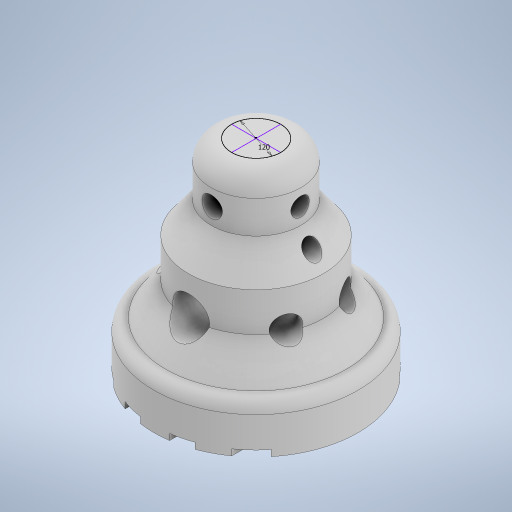
# Autodesk Inventor part: reef1
Saved by Autodesk Inventor 2024.3 (Build 283343000, 343)
## iProperties
Created: 2026-04-06
Part Number: reef1
Material: Genérico
Document SubType Name: Modeling
Designer: elena
Density: 1 g/cm^3
Appearance: Valor por defecto
Author: elena
Autodesk Inventor part; units mm, degrees
sketch "Boceto1" plane through (0, 0, 0) normal (0, 1, 0) x (-1, 0, 0)
  circle A0 centre (0, 0) radius 250
  dimension "d0" = 500
  constraints: 1 centre point, 1 coincident
  measures "d0" diameter of A0
extrude "Extrusión1" add sketch "Boceto1" along normal blind 100
sketch "Boceto2" plane through (0, 100, 0) normal (0, 1, 0) x (1, 0, 0)
  circle A0 centre (0, 0) radius 165
  dimension "d3" = 330
  constraints: 1 centre point, 1 coincident
  measures "d3" diameter of A0
extrude "Extrusión2" add sketch "Boceto2" along normal blind 175
chamfer "Chaflán1" distance 80 angle 35 1 edges at (-165, 100, 0) measured on face at (-165, 100.5, 0)
sketch "Boceto3" plane through (0, 275, 0) normal (0, 1, 0) x (1, 0, 0)
  point P0 (0, 0)
ref_plane "Plano de trabajo1" through (0, 350, 0) normal (0, 1, 0) x (1, 0, 0)
sketch "Boceto4" plane through (0, 350, 0) normal (0, 1, 0) x (1, 0, 0)
  circle A0 centre (0, 0) radius 110
  dimension "d10" = 220
  constraints: 1 centre point, 1 coincident
  measures "d10" diameter of A0
loft "Solevación1" add profiles "Boceto4" section 1 edges at (-165, 275, 0)
fillet "Empalme1" radius 30 1 edges at (250, 100, 0)
sketch "Boceto5" plane through (0, 350, 0) normal (0, 1, 0) x (1, 0, 0)
  circle A0 centre (0, 0) radius 110
  dimension "d16" = 220
  constraints: 1 centre point, 1 coincident
  measures "d16" diameter of A0
extrude "Extrusión3" add sketch "Boceto5" along normal blind 130
fillet "Empalme2" radius 50 1 edges at (-110, 480, 0)
sketch "Boceto6" plane through (0, 0, 0) normal (0, -1, 0) x (1, 0, 0)
  circle A0 centre (0, 0) radius 250
  dimension "d20" = 500
  constraints: 1 centre point, 1 coincident
  measures "d20" diameter of A0
extrude "Extrusión4" add sketch "Boceto6" along normal blind 20
sketch "Boceto7" plane through (0, 480, 0) normal (0, 1, 0) x (1, 0, 0)
  line L0 (-60.1732, 0) -> (60, 0)
  circle A0 centre (0, 0) radius 60 projected
  constraints: 2 end point, 1 horizontal, 1 horizontal alignment, 1 other
ref_plane "Plano de trabajo2" through (-60.1732, 480, 0) normal (0, 0, 1) x (1, 0, 0)
sketch "Boceto8" plane through (-60.1732, 480, 0) normal (0, 0, 1) x (1, 0, 0)
  point P0 (60.1732, -480)
sketch "Boceto9" plane through (0, -20, 0) normal (0, -1, 0) x (1, 0, 0)
  line L0 (0, 233.6633) -> (0, -235.8369)
  line L1 (-194.5383, 266.2675) -> (-194.5383, -277.679)
  line L2 (-194.5383, -277.679) -> (-144.5383, -277.679)
  line L3 (-144.5383, -277.679) -> (-144.5383, 266.2675)
  line L4 (-144.5383, 266.2675) -> (-194.5383, 266.2675)
  line L5 (-85.8577, 266.2675) -> (-85.8577, -277.679)
  line L6 (-85.8577, -277.679) -> (-35.8577, -277.679)
  line L7 (-35.8577, -277.679) -> (-35.8577, 266.2675)
  line L8 (-35.8577, 266.2675) -> (-85.8577, 266.2675)
  line L9 (194.5383, 266.2675) -> (194.5383, -277.679)
  line L10 (194.5383, -277.679) -> (144.5383, -277.679)
  line L11 (144.5383, -277.679) -> (144.5383, 266.2675)
  line L12 (144.5383, 266.2675) -> (194.5383, 266.2675)
  line L13 (85.8577, 266.2675) -> (85.8577, -277.679)
  line L14 (35.8577, -277.679) -> (35.8577, 266.2675)
  line L15 (85.8577, -277.679) -> (35.8577, -277.679)
  line L16 (35.8577, 266.2675) -> (85.8577, 266.2675)
  point P0 (0, 0)
  dimension "d24" = 50
  dimension "d25" = 50
  constraints: 34 end point, 8 symmetric about line, 4 perpendicular, 3 vertical, 2 horizontal
  measures "d24" distance of L1.end L2.end
  measures "d25" distance of L5.end L7.start
extrude "Extrusión5" cut sketch "Boceto9" against normal blind 15
sketch "Boceto10" plane through (-60.1732, 480, 0) normal (0, 0, 1) x (1, 0, 0)
  point P0 (60.1732, -480)
sketch "Boceto11" plane through (-60.1732, 480, 0) normal (0, 0, 1) x (1, 0, 0)
  circle A0 centre (60.1732, -292.5) radius 45
  point P0 (60.1732, -480)
  dimension "d28" = 90
  constraints: 1 centre point
  measures "d28" diameter of A0
extrude "Extrusión6" cut sketch "Boceto11" along normal mid plane 500
sketch "Boceto12" plane through (-60.1732, 480, 0) normal (0, 0, 1) x (1, 0, 0)
  line L0 (60.1732, -240.2586) -> (60.1732, -191.3822)
  line L1 (225.1732, -205) -> (-104.8268, -205) projected
  line L2 (225.1732, -300) -> (225.1732, -205) projected
  line L3 (225.1732, -300) -> (225.1732, -205)
  circle A0 centre (150.173, -292.5) radius 30
  line L4 (-104.8268, -300) -> (-104.8268, -205)
  circle A1 centre (-29.8267, -292.5) radius 30
  point P0 (60.1732, -480)
  dimension "d31" = 60
  constraints: 6 end point, 3 symmetric about line, 2 centre point, 2 point on line, 1 perpendicular, 1 other
  measures "d31" diameter of A0
revolve "Revolución1" cut sketch "Boceto12" angle 360 about axis through (-165, 180, 0) along (0, 1, 0) contours A1
revolve "Revolución2" cut sketch "Boceto12" angle 360 about axis through (165, 180, 0) along (0, 1, 0) contours A0
sketch "Boceto13" plane through (0, 480, 0) normal (0, 1, 0) x (1, 0, 0)
  circle A0 centre (0, 0) radius 60
  dimension "d34" = 120
  constraints: 1 centre point, 1 coincident
  measures "d34" diameter of A0
sketch "Boceto14" plane through (0, 480, 0) normal (0, 1, 0) x (1, 0, 0)
  circle A0 centre (0, 0) radius 60 projected
  line L0 (0, 60) -> (0, -60)
  constraints: 2 end point, 2 point on circle, 1 vertical
ref_plane "Plano de trabajo3" through (0, 480, -60) normal (-1, 0, 0) x (0, 0, 1)
sketch "Boceto15" plane through (-60.1732, 480, 0) normal (0, 0, 1) x (1, 0, 0)
  circle A0 centre (60.1732, -90) radius 25
  point P0 (60.1732, -480)
  dimension "d36" = 50
  constraints: 1 centre point
  measures "d36" diameter of A0
extrude "Extrusión7" cut sketch "Boceto15" along normal mid plane 500
sketch "Boceto16" plane through (0, 480, -60) normal (-1, 0, 0) x (0, 0, 1)
  circle A0 centre (60, -167.5) radius 20
  point P0 (60, -480)
  dimension "d39" = 40
  constraints: 1 centre point
  measures "d39" diameter of A0
extrude "Extrusión8" cut sketch "Boceto16" along normal mid plane 500
sketch "Boceto17" plane through (0, 480, -60) normal (-1, 0, 0) x (0, 0, 1)
  point P0 (60, -480)
ref_plane "Plano de trabajo4" through (-120, 480, -60) normal (-1, 0, 0) x (0, 0, 1)
sketch "Boceto18" plane through (-120, 480, -60) normal (-1, 0, 0) x (0, 0, 1)
  circle A0 centre (60, -90) radius 22.5
  point P0 (60, -480)
  dimension "d43" = 45
  constraints: 1 centre point
  measures "d43" diameter of A0
extrude "Extrusión9" cut sketch "Boceto18" against normal blind 60
ref_plane "Plano de trabajo5" through (120, 480, -60) normal (-1, 0, 0) x (0, 0, 1)
sketch "Boceto19" plane through (120, 480, -60) normal (-1, 0, 0) x (0, 0, 1)
  circle A0 centre (60, -90) radius 22.5 projected
  circle A1 centre (60, -90) radius 22.5
  point P0 (60, -480)
  constraints: 1 centre point, 1 coincident
extrude "Extrusión10" cut sketch "Boceto19" along normal blind 60
